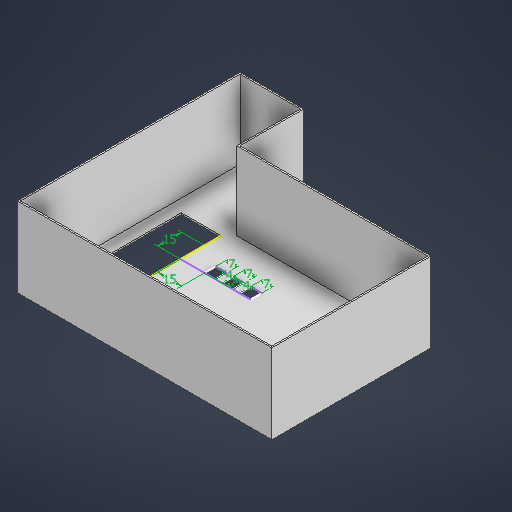
# Autodesk Inventor part: obudowatuner
Saved by Autodesk Inventor 2027 (Build 310192060, 192F)
## iProperties
Created: 2026-06-07
Part Number: obudowatuner
Material: Ogólny
Document SubType Name: Modeling
Designer: olab8
Density: 1 g/cm^3
Appearance: Domyślna
Author: olab8
Autodesk Inventor part; units mm, degrees
ref_plane "YZ Plane" through (0, 0, 0) normal (1, 0, 0) x (0, 1, 0)
ref_plane "XZ Plane" through (0, 0, 0) normal (0, 1, 0) x (-1, 0, 0)
ref_plane "XY Plane" through (0, 0, 0) normal (0, 0, 1) x (1, 0, 0)
sketch "Szkic1" plane through (0, 0, 0) normal (0, 1, 0) x (-1, 0, 0)
  line L0 (-25.3033, -19.9346) -> (-145.3033, -19.9346)
  line L1 (-145.3033, -19.9346) -> (-145.3033, 80.0654)
  line L2 (-145.3033, 80.0654) -> (14.6967, 80.0654)
  line L3 (14.6967, 80.0654) -> (14.6967, -19.9346)
  line L4 (-25.3033, -19.9346) -> (-25.3033, -59.9346)
  line L5 (14.6967, -59.9346) -> (14.6967, -19.9346)
  line L6 (-1.3707, 111.6296) -> (-1.3707, 118.6296)
  line L7 (-1.3707, 118.6296) -> (-30.3707, 118.6296)
  line L8 (-30.3707, 118.6296) -> (-30.3707, 111.6296)
  line L9 (-1.3707, 111.6296) -> (-30.3707, 111.6296)
  line L10 (14.6967, -59.9346) -> (-25.3033, -59.9346)
  point P0 (0, 0)
  dimension "d0" = 160
  dimension "d1" = 100
  dimension "d2" = 40
  dimension "d3" = 40
  dimension "d9" = 7
  dimension "d39" = 100
  constraints: 22 end point, 3 horizontal, 3 parallel, 2 perpendicular, 1 vertical
  measures "d0" distance of L1.end L2.end
  measures "d1" distance of L3.end L2.end
  measures "d2" distance of L5.start L3.end
  measures "d3" distance of L4.end L5.start
  measures "d9" distance of L6.start L6.end
  measures "d39" distance of L0.end L1.end
extrude "Wyciągnięcie proste1" add sketch "Szkic1" along normal blind 50 contours L0 L1 L2 L3 L5 L10 L4
shell "Skorupa1" thickness 1 removed faces 1 at (51.9699, 50, 46.732)
sketch "Szkic2" plane through (-13.6967, 1, -58.9346) normal (0, 0, 1) x (1, 0, 0)
  line L0 (-1, -1) -> (-1, 49) projected
  line L1 (39, -1) -> (39, 49) projected
  line L2 (-1, -1) -> (39, -1)
  line L3 (39, -1) -> (39, 36)
  line L4 (39, 36) -> (4.775, 36)
  line L5 (4.775, 36) -> (39, -1)
  line L6 (-1, -1) -> (39, 36)
  point P0 (13.6967, -1)
  point P1 (19, 17.5)
  dimension "d20" = 37
  constraints: 10 end point, 3 perpendicular, 1 midpoint, 1 point on line
  measures "d20" distance of L1.start L3.end
hole "Otwór1" at (5.3033, 18.5, -58.9346) direction (0, 0, -1) diameter 7 end through all
sketch "Szkic3" plane through (-13.6967, 1, 79.0654) normal (0, 1, 0) x (1, 0, 0)
  line L0 (158, 98) -> (38, 98) projected
  line L1 (38, 98) -> (0, 98)
  line L2 (0, 0) -> (0, 138) projected
  line L3 (0, 98) -> (1, 98)
  line L4 (0, 93.0725) -> (8, 93.0725)
  line L5 (8, 93.0725) -> (8, 20.0725)
  line L6 (8, 20.0725) -> (33, 20.0725)
  line L7 (33, 20.0725) -> (33, 93.0725)
  line L8 (33, 93.0725) -> (8, 93.0725)
  line L9 (8, 20.0725) -> (8, 0.0725)
  dimension "d41" = 73
  dimension "d42" = 25
  dimension "d43" = 20
  constraints: 16 end point, 4 perpendicular, 3 horizontal, 3 point on line
  measures "d41" distance of L4.end L5.end
  measures "d42" distance of L5.end L6.end
  measures "d43" distance of L5.end L9.end
extrude "Wyciągnięcie proste2" cut sketch "Szkic3" against normal blind 10
sketch "Szkic4" plane through (-13.6967, 1, 79.0654) normal (0, 1, 0) x (1, 0, 0)
  line L0 (33, 20.0725) -> (33, 93.0725) projected
  line L1 (33, 82.5783) -> (33, 67.5783)
  line L2 (33, 67.5783) -> (48, 67.5783)
  line L3 (48, 67.5783) -> (48, 74.5783)
  line L4 (48, 67.5783) -> (55, 67.5783)
  line L5 (55, 67.5783) -> (55, 74.5783)
  line L6 (55, 74.5783) -> (48, 74.5783)
  line L7 (48, 74.5783) -> (48, 67.5783)
  line L8 (55, 67.5783) -> (59, 67.5783)
  line L9 (59, 67.5783) -> (59, 74.5783)
  line L10 (59, 74.5783) -> (66, 74.5783)
  line L11 (66, 74.5783) -> (66, 67.5783)
  line L12 (66, 67.5783) -> (59, 67.5783)
  line L13 (66, 67.5783) -> (70, 67.5783)
  line L14 (70, 67.5783) -> (70, 74.5783)
  line L15 (70, 74.5783) -> (77, 74.5783)
  line L16 (77, 74.5783) -> (77, 67.5783)
  line L17 (77, 67.5783) -> (70, 67.5783)
  point P0 (48, 74.5783)
  dimension "d46" = 15
  dimension "d47" = 15
  dimension "d48" = 7
  dimension "d49" = 7
  dimension "d50" = 4
  dimension "d51" = 7
  dimension "d52" = 4
  dimension "d53" = 7
  constraints: 34 end point, 10 perpendicular, 7 point on line, 2 horizontal, 2 parallel
  measures "d46" distance of L1.start L1.end
  measures "d47" distance of L1.end L2.end
  measures "d48" distance of L2.end L3.end
  measures "d49" distance of L6.end L5.end
  measures "d50" distance of L4.end L8.end
  measures "d51" distance of L9.end L10.end
  measures "d52" distance of L11.end L13.end
  measures "d53" distance of L14.end L15.end
extrude "Wyciągnięcie proste3" cut sketch "Szkic4" against normal blind 10 contours L3 L6 L5 L4
extrude "Wyciągnięcie proste4" cut sketch "Szkic4" against normal blind 10 contours L14 L15 L16 L17 | L9 L10 L11 L12
